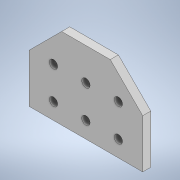
# Autodesk Inventor part: 3.5x2.5
Saved by Autodesk Inventor 2020 (Build 240168000, 168)
## iProperties
Created: 2020-01-14
Part Number: 3.5x2.5
Material: Generic
Document SubType Name: Modeling
Designer: 339294
Density: 1 g/cm^3
Appearance: Default
Author: 339294
Autodesk Inventor part; units mm, degrees
ref_plane "YZ Plane" through (0, 0, 0) normal (1, 0, 0) x (0, 1, 0)
ref_plane "XZ Plane" through (0, 0, 0) normal (0, 1, 0) x (-1, 0, 0)
ref_plane "XY Plane" through (0, 0, 0) normal (0, 0, 1) x (1, 0, 0)
sketch "Sketch1" plane through (0, 0, 0) normal (0, 0, 1) x (1, 0, 0)
  line L0 (0, 0) -> (63.5, 0)
  line L1 (63.5, 0) -> (63.5, 38.1)
  line L2 (38.1, 63.5) -> (0, 63.5)
  line L3 (-25.4, 38.1) -> (-25.4, 0)
  line L4 (-25.4, 0) -> (0, 0)
  line L5 (38.1, 63.5) -> (63.5, 38.1)
  line L6 (0, 63.5) -> (-25.4, 38.1)
  circle A0 centre (-6.35, 12.7) radius 3.2512
  circle A1 centre (-6.35, 38.1) radius 3.2512
  circle A2 centre (19.05, 38.1) radius 3.2512
  circle A3 centre (19.05, 12.7) radius 3.2512
  circle A4 centre (44.45, 38.1) radius 3.2512
  circle A5 centre (44.45, 12.7) radius 3.2512
  dimension "d5" = 63.5
  dimension "d6" = 25.4
  dimension "d7" = 38.1
  dimension "d8" = 25.4
  dimension "d9" = 25.4
  dimension "d10" = 38.1
  dimension "d11" = 25.4
  dimension "d12" = 25.4
  dimension "d13" = 38.1
  dimension "d14" = 135
  dimension "d15" = 135
  dimension "d16" = 90
  dimension "d17" = 6.5024
  dimension "d18" = 12.7
  dimension "d19" = 19.05
  dimension "d22" = 25.4
  dimension "d29" = 25.4
  constraints: 14 end point, 6 centre point, 2 horizontal, 1 perpendicular, 1 vertical, 10 other
  measures "d5" distance of L0.start L0.end
  measures "d6" distance of L3.end L4.end
  measures "d7" distance of L3.start L3.end
  measures "d8" horizontal distance of L2.end L3.start
  measures "d9" horizontal distance of L2.end L3.start
  measures "d10" distance of L2.start L2.end
  measures "d11" horizontal distance of L2.start L1.end
  measures "d12" horizontal distance of L2.start L1.end
  measures "d13" distance of L0.end L1.end
  measures "d14" angle of L2 L6
  measures "d15" angle of L3 L6
  measures "d16" angle of L3 L4
  measures "d17" diameter of A0
  measures "d18" distance from line of L4 A0.centre
  measures "d19" distance from line of L3 A0.centre
  measures "d22" distance of A0.centre A1.centre
  measures "d29" distance of A1.centre A2.centre
extrude "Extrusion1" add sketch "Sketch1" along normal blind 6.35
body "Solid1"
